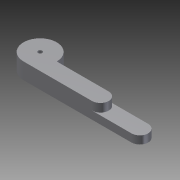
# Autodesk Inventor part: Traba
Saved by Autodesk Inventor 2011 (Build 150239000, 239)
## iProperties
Created: 2014-08-04
Part Number: Traba
Material: Por defecto
Document SubType Name: Chapa
Designer: amatiasq
Density: 1 g/cm^3
Sheet Metal Rule: Por defecto_mm
Author: amatiasq
Autodesk Inventor part; units mm, degrees
ref_plane "YZ Plane" through (0, 0, 0) normal (1, 0, 0) x (0, 1, 0)
ref_plane "XZ Plane" through (0, 0, 0) normal (0, 1, 0) x (-1, 0, 0)
ref_plane "XY Plane" through (0, 0, 0) normal (0, 0, 1) x (1, 0, 0)
sketch "Boceto1" plane through (0, 0, 0) normal (0, 0, 1) x (1, 0, 0)
  circle A0 centre (0, 0) radius 0.5
  arc A1 (4, 0) -> (0, -4) centre (0, 0) ccw
  line L0 (26, -4) -> (0, -4)
  arc A2 (26, -4) -> (26, 0) centre (26, -2) ccw
  line L1 (4, 0) -> (26, 0)
  dimension "d0" = 1
  dimension "d2" = 26
  constraints: 4 end point, 4 point on circle, 3 centre point, 2 coincident, 2 tangent, 1 horizontal, 1 parallel
  measures "d0" diameter of A0
  measures "d2" distance of L0.start L0.end
extrude "Extrusión1" add sketch "Boceto1" along normal blind 1.9
sketch "Boceto2" plane through (0, 0, 1.9) normal (0, 0, 1) x (1, 0, 0)
  circle A0 centre (0, 0) radius 0.5 projected
  arc A1 (4, 0) -> (0, -4) centre (0, 0) ccw projected
  line L0 (26, -4) -> (0, -4) projected
  line L1 (4, 0) -> (26, 0) projected
  arc A2 (16.5, -4) -> (16.5, 0) centre (16.5, -2) ccw
  line L2 (16.5, 0) -> (16.5, -4) construction
  line L3 (16.5, 0) -> (20.5, 0) construction
  dimension "d5" = 90
  constraints: 4 end point, 2 point on circle, 2 point on line, 2 tangent, 1 centre point, 1 horizontal, 1 perpendicular
  measures "d5" angle of L2 L3
extrude "Extrusión2" add sketch "Boceto2" along normal blind 2
equation "\"Radio_pliegue\" = Grosor"
equation "\"Anchura_desahogo_plegado\" = Grosor"
equation "\"Profundidad_desahogo_plegado\" = 0.5 * Grosor"
equation "\"Tamaño_destalonado\" = 4 * Grosor"
equation "\"Remanente_mínimo\" = 2 * Grosor"
equation "\"Radiodetransición\" = Radio_pliegue"
equation "\"Tamaño_de_radio_de_Jacobi\" = Radio_pliegue"
equation "\"TamañoSeparación\" = Grosor"
equation "\"Grosor\" = 0.5"
